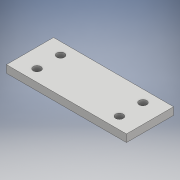
# Autodesk Inventor part: SPINDLE PLATE
Saved by Autodesk Inventor 2018 (Build 220112000, 112)
## iProperties
Created: 2018-10-16
Part Number: SPINDLE PLATE
Material: Generic
Document SubType Name: Modeling
Designer: Matthew Morey
Density: 1 g/cm^3
Appearance: Default
Author: Matthew Morey
Autodesk Inventor part; units mm, degrees
ref_plane "YZ Plane" through (0, 0, 0) normal (1, 0, 0) x (0, 1, 0)
ref_plane "XZ Plane" through (0, 0, 0) normal (0, 1, 0) x (-1, 0, 0)
ref_plane "XY Plane" through (0, 0, 0) normal (0, 0, 1) x (1, 0, 0)
sketch "Sketch1" plane through (0, 0, 0) normal (0, 0, 1) x (1, 0, 0)
  line L0 (-51, 20) -> (51, 20)
  line L1 (51, 20) -> (51, -20)
  line L2 (51, -20) -> (-51, -20)
  line L3 (-51, -20) -> (-51, 20)
  point P0 (0, 0)
  dimension "d0" = 102
  dimension "d1" = 51
  dimension "d2" = 40
  dimension "d3" = 20
  constraints: 8 end point, 2 parallel, 1 horizontal, 1 perpendicular
  measures "d0" distance of L0.start L0.end
  measures "d1" distance from line of point (0, 0) L1
  measures "d2" distance between parallel lines of L0 L2
  measures "d3" distance from line of point (0, 0) L0
extrude "Extrusion1" add sketch "Sketch1" along normal blind 6.35
sketch "Sketch3" plane through (0, 0, 0) normal (0, 0, -1) x (-1, 0, 0)
  circle A0 centre (-35, 10) radius 3.25
  circle A1 centre (-35, -10) radius 3.25
  circle A2 centre (35, -10) radius 3.25
  circle A3 centre (35, 10) radius 3.25
  line L0 (51, 20) -> (-51, 20) projected
  line L1 (-51, -20) -> (51, -20) projected
  line L2 (-51, 20) -> (-51, -20) projected
  line L3 (51, -20) -> (51, 20) projected
  point P0 (0, 0)
  dimension "d27" = 6.5
  dimension "d28" = 6.5
  dimension "d29" = 6.5
  dimension "d30" = 6.5
  dimension "d31" = 10
  dimension "d32" = 10
  dimension "d33" = 16
  dimension "d34" = 16
  dimension "d35" = 10
  dimension "d36" = 16
  dimension "d37" = 16
  dimension "d38" = 10
  constraints: 4 centre point
  measures "d27" diameter of A0
  measures "d28" diameter of A1
  measures "d29" diameter of A2
  measures "d30" diameter of A3
  measures "d31" distance from line of L0 A0.centre
  measures "d32" distance from line of L1 A1.centre
  measures "d33" distance from line of L2 A1.centre
  measures "d34" distance from line of L2 A0.centre
  measures "d35" distance from line of L0 A3.centre
  measures "d36" distance from line of L3 A3.centre
  measures "d37" distance from line of L3 A2.centre
  measures "d38" distance from line of L1 A2.centre
hole "Hole2" at (35, -10, 0) at (35, 10, 0) at (-35, 10, 0) at (-35, -10, 0) direction (0, 0, 1) diameter 6.5 end through all countersink diameter 8 countersink angle 90
body "Solid1"
